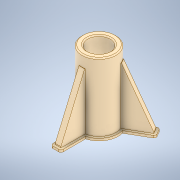
# Autodesk Inventor part: stojak
Saved by Autodesk Inventor 2021 (Build 250183000, 183)
## iProperties
Created: 2021-05-20
Part Number: stojak
Material: Polietylen, o małej gęstości
Document SubType Name: Modeling
Designer: Wojciech Wołczek
Density: 0.894 g/cm^3
Appearance: Gładki — w kolorze złamanej bieli
Mass: 31.0126 g
Surface Area: 158.451 cm^2
Volume: 34.6897 cm^3
Author: Wojciech Wołczek
Autodesk Inventor part; units mm, degrees
ref_plane "YZ Plane" through (0, 0, 0) normal (1, 0, 0) x (0, 1, 0)
ref_plane "XZ Plane" through (0, 0, 0) normal (0, 1, 0) x (-1, 0, 0)
ref_plane "XY Plane" through (0, 0, 0) normal (0, 0, 1) x (1, 0, 0)
sketch "Szkic1" plane through (0, 0, 0) normal (0, 1, 0) x (-1, 0, 0)
  circle A0 centre (0, 0) radius 10
  circle A1 centre (0, 0) radius 15
  dimension "d0" = 20
  dimension "d1" = 30
  constraints: 2 centre point, 2 coincident
  measures "d0" diameter of A0
  measures "d1" diameter of A1
extrude "Wyciągnięcie proste1" add sketch "Szkic1" along normal blind 60
sketch "Szkic2" plane through (0, 0, 0) normal (0, -1, 0) x (1, 0, 0)
  line L0 (2.5, 36.2128) -> (-2.5, 36.2128)
  line L1 (-2.5, 36.2128) -> (-2.5, 11.2128)
  line L2 (-2.5, 11.2128) -> (2.5, 11.2128)
  line L3 (2.5, 11.2128) -> (2.5, 36.2128)
  line L4 (2.5, 36.2128) -> (-2.5, 11.2128) construction
  line L5 (-2.5, 36.2128) -> (2.5, 11.2128) construction
  point P0 (0, 0)
  point P1 (0, 23.7128)
  dimension "d4" = 5
  dimension "d5" = 25
  constraints: 12 end point, 2 midpoint, 2 parallel, 1 horizontal, 1 perpendicular
  measures "d4" distance of L2.end L1.end
  measures "d5" distance of L1.end L0.end
extrude "Wyciągnięcie proste2" add sketch "Szkic2" against normal blind 50
chamfer "Faza1" distance 21 distance2 49 1 edges at (0, 50, 36.2128) measured on face at (-0.2789, 50, 29.1341)
pattern_circular "Szyk kołowy1" count 3 over 360 about axis through (0, 0, 0) along (0, 1, 0) of "Faza1", "Wyciągnięcie proste2"
sketch "Szkic3" plane through (0, 0, 0) normal (0, -1, 0) x (1, 0, 0)
  arc A0 (-11.5587, -9.5602) -> (11.5587, -9.5602) centre (0, 0) ccw projected
  line L0 (11.5587, -9.5602) -> (30.1112, -20.2715) projected
  line L1 (30.1112, -20.2715) -> (32.6112, -15.9413) projected
  line L2 (32.6112, -15.9413) -> (14.0587, -5.23) projected
  arc A1 (14.0587, -5.23) -> (2.5, 14.7902) centre (0, 0) ccw projected
  line L3 (2.5, 14.7902) -> (2.5, 36.2128) projected
  line L4 (2.5, 36.2128) -> (-2.5, 36.2128) projected
  line L5 (-2.5, 36.2128) -> (-2.5, 14.7902) projected
  arc A2 (-2.5, 14.7902) -> (-14.0587, -5.23) centre (0, 0) ccw projected
  line L6 (-14.0587, -5.23) -> (-32.6112, -15.9413) projected
  line L7 (-32.6112, -15.9413) -> (-30.1112, -20.2715) projected
  line L8 (-30.1112, -20.2715) -> (-11.5587, -9.5602) projected
  circle A3 centre (0, 0) radius 10 projected
  arc A4 (16.4473, -4.2997) -> (4.5, 16.3936) centre (0, 0) ccw
  line L9 (16.4473, -4.2997) -> (35.3433, -15.2093)
  line L10 (35.3433, -15.2093) -> (30.8433, -23.0035)
  line L11 (30.8433, -23.0035) -> (11.9473, -12.0939)
  arc A5 (-11.9473, -12.0939) -> (11.9473, -12.0939) centre (0, 0) ccw
  line L12 (-11.9473, -12.0939) -> (-30.8433, -23.0035)
  line L13 (-30.8433, -23.0035) -> (-35.3433, -15.2093)
  line L14 (-35.3433, -15.2093) -> (-16.4473, -4.2997)
  arc A6 (-4.5, 16.3936) -> (-16.4473, -4.2997) centre (0, 0) ccw
  line L15 (-4.5, 16.3936) -> (-4.5, 38.2128)
  line L16 (-4.5, 38.2128) -> (4.5, 38.2128)
  line L17 (4.5, 38.2128) -> (4.5, 16.3936)
  dimension "d14" = 2
  constraints: 18 end point, 6 point on circle, 3 centre point, 11 other
  measures "d14" radial gap between concentric circles of A1 A4
extrude "Wyciągnięcie proste3" add sketch "Szkic3" along normal blind 2 contours L8 L7 L6 A2 L5 L4 L3 A1 L2 L1 L0 A0 | A3 | L9 L10 L11 A5 L12 L13 L14 A6 L15 L16 L17 A4
fillet "Zaokrąglenie1" radius 2 6 edges at (35.3433, -1, -15.2093) (30.8433, -1, -23.0035) (-30.8433, -1, -23.0035) (-35.3433, -1, -15.2093) (-4.5, -1, 38.2128) (4.5, -1, 38.2128)
chamfer "Faza2" distance 1 angle 45 2 edges at (15, 60, 0) (10, 60, 0)
